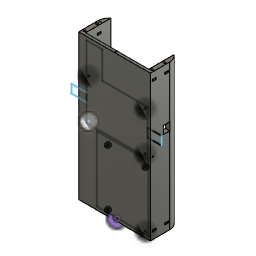
robottikoiran jetson runko v4 (Autodesk Fusion 360 design; units mm, degrees)
Autodesk Fusion 360 part; units mm, degrees
sketch "Sketch1" plane through (0, 0, 0) normal (0, 1, 0) x (1, 0, 0)
  line L0 (-48.5, 30) -> (-55, 30)
  line L1 (-55, 30) -> (-55, 0)
  line L2 (-55, 0) -> (0, 0)
  line L3 (0, 0) -> (0, 4)
  line L4 (0, 4) -> (-48.5, 4)
  line L5 (-48.5, 4) -> (-48.5, 30)
  line L6 (55, 30) -> (55, 0)
  line L7 (48.5, 4) -> (48.5, 30)
  line L8 (48.5, 30) -> (55, 30)
  line L9 (55, 0) -> (0, 0)
  line L10 (0, 4) -> (48.5, 4)
  dimension "d1" = 55
  dimension "d2" = 6.5
  dimension "d3" = 4
  dimension "d4" = 30
  constraint horizontal L0
  constraint perpendicular L0 L1
  constraint coincident L2.end L3.start
  constraint perpendicular L1 L2
  constraint perpendicular L2 L3
  constraint perpendicular L3 L4
  constraint perpendicular L0 L5
  constraint symmetric L0.start L3 L7.end
  constraint symmetric L0.end L3 L6.start
  constraint symmetric L1.end L3 L6.end
  constraint symmetric L2.end L3 L9.end
  constraint symmetric L4.start L3 L10.start
  constraint symmetric L3 L4.end L7.start
  measures "d1" distance of L1.end L2.end
  measures "d2" distance of L0.start L0.end
  measures "d3" distance of L2.end L3.end
  measures "d4" distance of L0 L2
extrude "Extrude1" add sketch "Sketch1" along normal blind 223
sketch "Sketch2" plane through (0, 223, 0) normal (0, 1, 0) x (-1, 0, 0)
  line L0 (48.5, -4) -> (48.5, -30)
  line L1 (48.5, -30) -> (55, -30)
  line L2 (55, -30) -> (55, 0)
  line L3 (55, 0) -> (-55, 0)
  line L4 (-55, 0) -> (-55, -30)
  line L5 (-55, -30) -> (-48.5, -30)
  line L6 (-48.5, -30) -> (-48.5, -4)
  line L7 (-48.5, -4) -> (48.5, -4)
  circle A0 centre (51.75, -25) radius 1.6
  circle A1 centre (51.75, -6) radius 1.6
  line L8 (0, 1.75) -> (0, 22.5)
  circle A2 centre (-51.75, -25) radius 1.6
  circle A3 centre (-51.75, -6) radius 1.6
  point P0 (-51.75, -6)
  point P1 (-51.75, -25)
  dimension "d7" = 3.2
  dimension "d8" = 3.2
  dimension "d9" = 19
  dimension "d10" = 5
  dimension "d11" = 3.25
  constraint symmetric A0.centre L8 P1
  constraint symmetric A1.centre L8 P0
  constraint symmetric A0 L8 A2
  constraint symmetric A1 L8 A3
  measures "d7" diameter of A0
  measures "d8" diameter of A1
  measures "d9" distance of A0.centre A1.centre
  measures "d10" distance of L1 A0.centre
  measures "d11" distance of L0 A0.centre
extrude "Extrude2" cut sketch "Sketch2" against normal blind 15 contours A0 | A1 | A2 | A3
sketch "Sketch3" plane through (0, 0, 0) normal (0, 1, 0) x (-1, 0, 0)
  circle A0 centre (51.75, -6) radius 1.6
  circle A1 centre (51.75, -25) radius 1.6
  line L0 (48.5, -30) -> (55, -30)
  line L1 (48.5, -4) -> (48.5, -30)
  line L2 (0, 1.75) -> (0, 22.5)
  circle A2 centre (-51.75, -25) radius 1.6
  circle A3 centre (-51.75, -6) radius 1.6
  line L3 (48.5, -30) -> (48.5, -4)
  line L4 (48.5, -4) -> (-48.5, -4)
  line L5 (-48.5, -4) -> (-48.5, -30)
  line L6 (-48.5, -30) -> (-55, -30)
  line L7 (-55, -30) -> (-55, 0)
  line L8 (-55, 0) -> (55, 0)
  line L9 (55, 0) -> (55, -30)
  line L10 (55, -30) -> (48.5, -30)
  dimension "d14" = 3.2
  dimension "d15" = 3.2
  dimension "d16" = 19
  dimension "d17" = 5
  dimension "d18" = 3.25
  constraint symmetric A0 L2 A3
  constraint symmetric A1 L2 A2
  measures "d14" diameter of A0
  measures "d15" diameter of A1
  measures "d16" distance of A0.centre A1.centre
  measures "d17" distance of A1.centre L0
  measures "d18" distance of A1.centre L1
extrude "Extrude3" cut sketch "Sketch3" along normal blind 15 contours A0 | A1 | A2 | A3
sketch "Sketch4" plane through (55, 0, 0) normal (1, 0, 0) x (0, 0, -1)
  line L0 (0, 0) -> (30, 0)
  line L1 (30, 0) -> (30, 223)
  line L2 (30, 223) -> (0, 223)
  line L3 (0, 223) -> (0, 0)
  line L4 (22.2, 213) -> (27.8, 213)
  line L5 (27.8, 213) -> (27.8, 210.2)
  line L6 (27.8, 210.2) -> (22.2, 210.2)
  line L7 (22.2, 210.2) -> (22.2, 213)
  line L8 (8.8, 213) -> (3.2, 213)
  line L9 (3.2, 213) -> (3.2, 210.2)
  line L10 (3.2, 210.2) -> (8.8, 210.2)
  line L11 (8.8, 210.2) -> (8.8, 213)
  line L12 (-42.9393, 111.5) -> (70.6, 111.5)
  line L13 (27.8, 12.8) -> (22.2, 12.8)
  line L14 (8.8, 12.8) -> (8.8, 10)
  line L15 (22.2, 10) -> (27.8, 10)
  line L16 (27.8, 10) -> (27.8, 12.8)
  line L17 (3.2, 10) -> (3.2, 12.8)
  line L18 (3.2, 12.8) -> (8.8, 12.8)
  line L19 (8.8, 10) -> (3.2, 10)
  line L20 (22.2, 12.8) -> (22.2, 10)
  dimension "d21" = 19
  dimension "d22" = 10
  dimension "d23" = 5.6
  dimension "d24" = 5.6
  dimension "d25" = 10
  dimension "d26" = 2.2
  dimension "d27" = 111.5
  dimension "d41" = 2.8
  dimension "d42" = 2.8
  constraint horizontal L4
  constraint vertical L5
  constraint horizontal L6
  constraint vertical L7
  constraint horizontal L8
  constraint vertical L9
  constraint horizontal L10
  constraint vertical L11
  constraint perpendicular L1 L12
  constraint symmetric L4.start L12 L15.start
  constraint symmetric L4.end L12 L15.end
  constraint symmetric L5.end L12 L13.start
  constraint symmetric L6.end L12 L13.end
  constraint symmetric L8.start L12 L14.end
  constraint symmetric L8.end L12 L17.start
  constraint symmetric L9.end L12 L17.end
  constraint symmetric L10.end L12 L14.start
  measures "d21" distance of L4.end L8.start
  measures "d22" distance of L2 L4
  measures "d23" distance of L5.end L6.end
  measures "d24" distance of L9.end L10.end
  measures "d25" distance of L2 L8
  measures "d26" distance of L1 L5
  measures "d27" distance of L2 L12
  measures "d41" distance of L8.start L10.end
  measures "d42" distance of L4.end L5.end
extrude "Extrude4" cut sketch "Sketch4" against normal blind 6.5 contours L4 L5 L6 L7 | L8 L9 L10 L11 | L13 L15 L16 L20 | L14 L17 L18 L19
sketch "Sketch5" plane through (-55, 0, 0) normal (-1, 0, 0) x (0, 0, 1)
  line L0 (-30, 0) -> (0, 0)
  line L1 (0, 0) -> (0, 223)
  line L2 (0, 223) -> (-30, 223)
  line L3 (-30, 223) -> (-30, 0)
  line L4 (-22.2, 10) -> (-27.8, 10)
  line L5 (-27.8, 10) -> (-27.8, 12.8)
  line L6 (-27.8, 12.8) -> (-22.2, 12.8)
  line L7 (-22.2, 12.8) -> (-22.2, 10)
  line L8 (-3.2, 10) -> (-8.8, 10)
  line L9 (-8.8, 10) -> (-8.8, 12.8)
  line L10 (-8.8, 12.8) -> (-3.2, 12.8)
  line L11 (-3.2, 12.8) -> (-3.2, 10)
  line L12 (28.3508, 111.5) -> (-44.2401, 111.5)
  line L13 (-27.8, 213) -> (-27.8, 210.2)
  line L14 (-22.2, 213) -> (-27.8, 213)
  line L15 (-27.8, 210.2) -> (-22.2, 210.2)
  line L16 (-22.2, 210.2) -> (-22.2, 213)
  line L17 (-8.8, 210.2) -> (-3.2, 210.2)
  line L18 (-3.2, 210.2) -> (-3.2, 213)
  line L19 (-3.2, 213) -> (-8.8, 213)
  line L20 (-8.8, 213) -> (-8.8, 210.2)
  dimension "d30" = 19
  dimension "d31" = 5.6
  dimension "d32" = 5.6
  dimension "d33" = 2.2
  dimension "d34" = 10
  dimension "d35" = 10
  dimension "d36" = 2.8
  dimension "d37" = 2.8
  dimension "d38" = 111.5
  constraint horizontal L4
  constraint vertical L5
  constraint horizontal L6
  constraint vertical L7
  constraint horizontal L8
  constraint vertical L9
  constraint horizontal L10
  constraint vertical L11
  constraint perpendicular L1 L12
  constraint symmetric L4.start L12 L14.start
  constraint symmetric L4.end L12 L13.start
  constraint symmetric L5.end L12 L13.end
  constraint symmetric L6.end L12 L15.end
  constraint symmetric L8.start L12 L18.end
  constraint symmetric L8.end L12 L19.end
  constraint symmetric L9.end L12 L17.start
  constraint symmetric L10.end L12 L17.end
  measures "d30" distance of L4.end L8.end
  measures "d31" distance of L4.start L4.end
  measures "d32" distance of L8.start L8.end
  measures "d33" distance of L3 L4.end
  measures "d34" distance of L0 L4
  measures "d35" distance of L0 L8
  measures "d36" distance of L8.end L9.end
  measures "d37" distance of L4.start L6.end
  measures "d38" distance of L0 L12
extrude "Extrude5" cut sketch "Sketch5" against normal blind 6.5 contours L4 L5 L6 L7 | L8 L9 L10 L11 | L13 L14 L15 L16 | L17 L18 L19 L20
sketch "Sketch6" plane through (0, 0, -4) normal (0, 0, -1) x (-1, 0, 0)
  line L0 (-48.5, 0) -> (48.5, 0)
  line L1 (48.5, 0) -> (48.5, 10)
  line L2 (48.5, 10) -> (48.5, 12.8)
  line L3 (48.5, 12.8) -> (48.5, 210.2)
  line L4 (48.5, 210.2) -> (48.5, 213)
  line L5 (48.5, 213) -> (48.5, 223)
  line L6 (48.5, 223) -> (-48.5, 223)
  line L7 (-48.5, 223) -> (-48.5, 213)
  line L8 (-48.5, 213) -> (-48.5, 210.2)
  line L9 (-48.5, 210.2) -> (-48.5, 12.8)
  line L10 (-48.5, 12.8) -> (-48.5, 10)
  line L11 (-48.5, 10) -> (-48.5, 0)
  line L12 (31, 1) -> (-48, 1)
  line L13 (-48, 1) -> (-48, 101)
  line L14 (-48, 101) -> (31, 101)
  line L15 (31, 101) -> (31, 1)
  circle A0 centre (-44, 5) radius 1.375
  circle A1 centre (14, 5) radius 1.375
  circle A2 centre (14, 91) radius 1.375
  circle A3 centre (-44, 91) radius 1.375
  line L16 (-47, 104) -> (47, 104)
  line L17 (47, 104) -> (47, 213.6)
  line L18 (47, 213.6) -> (22.8, 213.6)
  line L19 (22.8, 213.6) -> (22.8, 172)
  line L20 (22.8, 172) -> (-47, 172)
  line L21 (-47, 172) -> (-47, 104)
  circle A4 centre (-43.45, 107.8) radius 1
  circle A5 centre (43.2, 107.8) radius 1
  circle A6 centre (-43.5, 168.4) radius 1
  circle A7 centre (43.3, 168.3) radius 1
  line L22 (-47, 131.4) -> (-68.4121, 131.4)
  line L23 (-68.4121, 131.4) -> (-68.4121, 144.4)
  line L24 (-68.4121, 144.4) -> (-47, 144.4)
  line L25 (-47, 144.4) -> (-47, 131.4)
  line L26 (47, 131.4) -> (70, 131.4)
  line L27 (70, 131.4) -> (70, 144.4)
  line L28 (70, 144.4) -> (47, 144.4)
  line L29 (47, 144.4) -> (47, 131.4)
  point P0 (14, 5)
  point P1 (-44, 91)
  point P2 (14, 91)
  dimension "d43" = 100
  dimension "d44" = 79
  dimension "d48" = 2.75
  dimension "d49" = 4
  dimension "d50" = 4
  dimension "d53" = 58
  dimension "d54" = 86
  dimension "d55" = 2.75
  dimension "d56" = 2.75
  dimension "d57" = 2.75
  dimension "d58" = 94
  dimension "d59" = 109.6
  dimension "d60" = 68
  dimension "d61" = 24.2
  dimension "d62" = 47
  dimension "d63" = 48
  dimension "d64" = 1
  dimension "d65" = 3
  dimension "d66" = 2
  dimension "d67" = 3.55
  dimension "d68" = 3.8
  dimension "d69" = 2
  dimension "d70" = 3.8
  dimension "d71" = 2
  dimension "d72" = 3.5
  dimension "d73" = 3.6
  dimension "d74" = 64.3
  dimension "d75" = 3.7
  dimension "d76" = 2
  dimension "d77" = 13
  dimension "d78" = 27.4
  dimension "d79" = 13
  constraint horizontal L12
  constraint vertical L13
  constraint horizontal L14
  constraint vertical L15
  constraint coincident P0 A1.centre
  constraint coincident P2 A2.centre
  constraint coincident P1 A3.centre
  constraint perpendicular L15 L16
  constraint perpendicular L14 L17
  constraint perpendicular L17 L18
  constraint perpendicular L18 L19
  constraint perpendicular L19 L20
  constraint perpendicular L16 L21
  constraint horizontal L22
  constraint vertical L23
  constraint horizontal L24
  constraint vertical L25
  constraint coincident L21 L22.start
  constraint horizontal L26
  constraint vertical L27
  constraint horizontal L28
  constraint vertical L29
  constraint coincident L17 L26.start
  measures "d43" distance of L12.start L14.end
  measures "d44" distance of L12.start L12.end
  measures "d48" diameter of A0
  measures "d49" distance of L12 A0.centre
  measures "d50" distance of L13 A0.centre
  measures "d55" diameter of A1
  measures "d56" diameter of A2
  measures "d57" diameter of A3
  measures "d58" distance of L16.start L16.end
  measures "d59" distance of L16 L18
  measures "d60" distance of L16.start L20.end
  measures "d61" distance of L17.end L18.end
  measures "d62" distance of origin L21
  measures "d63" distance of origin L13
  measures "d64" distance of origin L12
  measures "d65" distance of L14 L16
  measures "d66" diameter of A4
  measures "d67" distance of L21 A4.centre
  measures "d68" distance of L16 A4.centre
  measures "d69" diameter of A5
  measures "d70" distance of L17 A5.centre
  measures "d71" diameter of A6
  measures "d72" distance of L21 A6.centre
  measures "d73" distance of L20 A6.centre
  measures "d74" distance of L16 A7.centre
  measures "d75" distance of L17 A7.centre
  measures "d76" diameter of A7
  measures "d77" distance of L22.end L23.end
  measures "d78" distance of L16 L22
  measures "d79" distance of L26.start L28.end
hole "Hole1" at (-14, 5, -4) at (-14, 91, -4) at (-43.2, 107.8, -4) at (-43.3, 168.3, -4) at (43.5, 168.4, -4) at (43.45, 107.8, -4) at (44, 91, -4) at (44, 5, -4) direction (0, 0, 1) diameter 1 depth 8 tip angle 118
sketch "Sketch7" plane through (-55, 0, 0) normal (-1, 0, 0) x (0, 0, 1)
  line L0 (-27.8, 10) -> (-27.8, 12.8)
  line L1 (-27.8, 12.8) -> (-22.2, 12.8)
  line L2 (-22.2, 12.8) -> (-22.2, 10)
  line L3 (-22.2, 10) -> (-27.8, 10)
  line L4 (-3.2, 210.2) -> (-8.8, 210.2)
  line L5 (-8.8, 210.2) -> (-8.8, 213)
  line L6 (-8.8, 213) -> (-3.2, 213)
  line L7 (-3.2, 213) -> (-3.2, 210.2)
  line L8 (-8.8, 10) -> (-8.8, 12.8)
  line L9 (-8.8, 12.8) -> (-3.2, 12.8)
  line L10 (-3.2, 12.8) -> (-3.2, 10)
  line L11 (-3.2, 10) -> (-8.8, 10)
  line L12 (-27.8, 213) -> (-22.2, 213)
  line L13 (-22.2, 213) -> (-22.2, 210.2)
  line L14 (-22.2, 210.2) -> (-27.8, 210.2)
  line L15 (-27.8, 210.2) -> (-27.8, 213)
  line L16 (-30, 0) -> (0, 0)
  line L17 (0, 0) -> (0, 223)
  line L18 (0, 223) -> (-30, 223)
  line L19 (-30, 223) -> (-30, 0)
  circle A0 centre (-4, 109.925) radius 1
  line L20 (-35, 143.4) -> (-20, 143.4)
  line L21 (-20, 143.4) -> (-20, 131.4)
  line L22 (-20, 131.4) -> (-35, 131.4)
  line L23 (-35, 131.4) -> (-35, 143.4)
  circle A1 centre (-17, 7) radius 4
  line L24 (-28, 53) -> (-10, 53)
  line L25 (-10, 53) -> (-10, 34)
  line L26 (-10, 34) -> (-28, 34)
  line L27 (-28, 34) -> (-28, 53)
  line L28 (-16, 99) -> (-9, 99)
  line L29 (-9, 99) -> (-9, 87)
  line L30 (-9, 87) -> (-16, 87)
  line L31 (-16, 87) -> (-16, 99)
  line L32 (-14.7213, 34) -> (-15, 34)
  line L33 (-15, 34) -> (-15, 0)
  line L34 (-15, 0) -> (-14.7213, 0)
  line L35 (-14.7213, 0) -> (-14.7213, 34)
  point P0 (-4, 131.4)
  dimension "d83" = 2
  dimension "d84" = 109.925
  dimension "d85" = 26
  dimension "d86" = 12
  dimension "d89" = 131.4
  dimension "d90" = 15
  dimension "d91" = 10
  dimension "d92" = 8
  dimension "d93" = 13
  dimension "d94" = 7
  dimension "d95" = 19
  dimension "d96" = 18
  dimension "d97" = 20
  dimension "d98" = 34
  dimension "d99" = 12
  dimension "d100" = 7
  dimension "d101" = 21
  dimension "d102" = 87
  constraint horizontal L20
  constraint vertical L21
  constraint horizontal L22
  constraint vertical L23
  constraint horizontal L24
  constraint vertical L25
  constraint horizontal L26
  constraint vertical L27
  constraint horizontal L28
  constraint vertical L29
  constraint horizontal L30
  constraint vertical L31
  constraint horizontal L32
  constraint vertical L33
  constraint horizontal L34
  constraint vertical L35
  constraint midpoint L16 L33.end
  constraint coincident L26 L32.start
  measures "d83" diameter of A0
  measures "d84" distance of L16 A0.centre
  measures "d85" distance of L19 A0.centre
  measures "d86" distance of L20.end L21.end
  measures "d89" distance of L16 L22
  measures "d90" distance of L21.end L22.end
  measures "d91" distance of L19 L21
  measures "d92" diameter of A1
  measures "d93" distance of L19 A1.centre
  measures "d94" distance of L16 A1.centre
  measures "d95" distance of L24.start L26.end
  measures "d96" distance of L24.start L24.end
  measures "d97" distance of L19 L25
  measures "d98" distance of L16 L26
  measures "d99" distance of L28.start L30.end
  measures "d100" distance of L29.end L30.end
  measures "d101" distance of L19 L29
  measures "d102" distance of L16 L30
extrude "Extrude6" cut sketch "Sketch7" against normal blind 6.8 contours L19 L20 L21 L22 | A1 L33 L35 | A1 L33 | A1 L35 | L24 L25 L26 L27 L32 | A0 | L28 L29 L30 L31
sketch "Sketch8" plane through (55, 0, 0) normal (1, 0, 0) x (0, 0, -1)
  line L0 (27.8, 213) -> (27.8, 210.2)
  line L1 (27.8, 210.2) -> (22.2, 210.2)
  line L2 (22.2, 210.2) -> (22.2, 213)
  line L3 (22.2, 213) -> (27.8, 213)
  line L4 (3.2, 12.8) -> (8.8, 12.8)
  line L5 (8.8, 12.8) -> (8.8, 10)
  line L6 (8.8, 10) -> (3.2, 10)
  line L7 (3.2, 10) -> (3.2, 12.8)
  line L8 (3.2, 213) -> (8.8, 213)
  line L9 (8.8, 213) -> (8.8, 210.2)
  line L10 (8.8, 210.2) -> (3.2, 210.2)
  line L11 (3.2, 210.2) -> (3.2, 213)
  line L12 (27.8, 10) -> (22.2, 10)
  line L13 (22.2, 10) -> (22.2, 12.8)
  line L14 (22.2, 12.8) -> (27.8, 12.8)
  line L15 (27.8, 12.8) -> (27.8, 10)
  line L16 (0, 0) -> (30, 0)
  line L17 (30, 0) -> (30, 223)
  line L18 (30, 223) -> (0, 223)
  line L19 (0, 223) -> (0, 0)
  circle A0 centre (4, 109.925) radius 1
  line L20 (30, 131.4) -> (20, 131.4)
  line L21 (20, 143.4) -> (35, 143.4)
  line L22 (35, 143.4) -> (35, 131.4)
  line L23 (35, 131.4) -> (20, 131.4)
  line L24 (20, 131.4) -> (20, 143.4)
  dimension "d105" = 2
  dimension "d106" = 26
  dimension "d107" = 109.925
  dimension "d109" = 15
  dimension "d110" = 12
  dimension "d111" = 131.4
  dimension "d112" = 10
  constraint horizontal L21
  constraint vertical L22
  constraint horizontal L23
  constraint vertical L24
  measures "d105" diameter of A0
  measures "d106" distance of L17 A0.centre
  measures "d107" distance of L16 A0.centre
  measures "d109" distance of L21.start L21.end
  measures "d110" distance of L21.end L22.end
  measures "d111" distance of L16 L23
  measures "d112" distance of L17 L24
extrude "Extrude7" cut sketch "Sketch8" against normal blind 6.8 contours L17 L20 L21 L23 L24 | A0
sketch "Sketch9" plane through (0, 0, 0) normal (0, -1, 0) x (1, 0, 0)
  circle A0 centre (-51.75, -6) radius 1.6
  circle A1 centre (51.75, -6) radius 1.6
  circle A2 centre (-51.75, -25) radius 1.6
  circle A3 centre (51.75, -25) radius 1.6
  line L0 (-48.5, -30) -> (-48.5, -4)
  line L1 (-48.5, -4) -> (48.5, -4)
  line L2 (48.5, -4) -> (48.5, -30)
  line L3 (48.5, -30) -> (55, -30)
  line L4 (55, -30) -> (55, 0)
  line L5 (55, 0) -> (-55, 0)
  line L6 (-55, 0) -> (-55, -30)
  line L7 (-55, -30) -> (-48.5, -30)
  circle A4 centre (0, -2) radius 1
  point P0 (0, -4)
  dimension "d115" = 2
  dimension "d116" = 2
  measures "d115" diameter of A4
  measures "d116" distance of A4.centre P0
extrude "Extrude8" cut sketch "Sketch9" against normal blind 8 contours A4
sketch "Sketch10" plane through (0, 223, 0) normal (0, 1, 0) x (-1, 0, 0)
  circle A0 centre (51.75, -6) radius 1.6
  circle A1 centre (-51.75, -6) radius 1.6
  circle A2 centre (51.75, -25) radius 1.6
  circle A3 centre (-51.75, -25) radius 1.6
  line L0 (48.5, -4) -> (48.5, -30)
  line L1 (48.5, -30) -> (55, -30)
  line L2 (55, -30) -> (55, 0)
  line L3 (55, 0) -> (-55, 0)
  line L4 (-55, 0) -> (-55, -30)
  line L5 (-55, -30) -> (-48.5, -30)
  line L6 (-48.5, -30) -> (-48.5, -4)
  line L7 (-48.5, -4) -> (48.5, -4)
  circle A4 centre (0, -2) radius 1
  point P0 (0, -4)
  dimension "d119" = 2
  dimension "d120" = 2
  measures "d119" diameter of A4
  measures "d120" distance of A4.centre P0
extrude "Extrude9" cut sketch "Sketch10" against normal blind 8 contours A4
sketch "Sketch11" plane through (0, 0, -4) normal (0, 0, -1) x (-1, 0, 0)
sketch "Sketch12" plane through (0, 0, -30) normal (0, 0, -1) x (-1, 0, 0)
  line L0 (55, 131.4) -> (48.5, 131.4)
  line L1 (48.5, 131.4) -> (48.5, 0)
  line L2 (48.5, 0) -> (55, 0)
  line L3 (55, 0) -> (55, 131.4)
  line L4 (-55, 223) -> (-48.5, 223)
  line L5 (-48.5, 223) -> (-48.5, 0)
  line L6 (-48.5, 0) -> (-55, 0)
  line L7 (-55, 0) -> (-55, 223)
  line L8 (48.5, 0) -> (55, 0)
  line L9 (55, 0) -> (55, 223.0049)
  line L10 (55, 223.0049) -> (48.5, 223.0049)
  line L11 (48.5, 223.0049) -> (48.5, 0)
  constraint horizontal L4
  constraint vertical L5
  constraint horizontal L6
  constraint vertical L7
  constraint horizontal L8
  constraint vertical L9
  constraint horizontal L10
  constraint vertical L11
  constraint coincident L1.end L2.start
extrude "Extrude10" add sketch "Sketch12" along normal blind 13
fillet "Fillet1" radius 17 2 edges at (-55, 111.5024, -43) (55, 111.5, -43)
